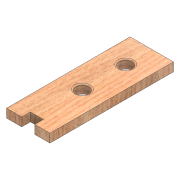
# Autodesk Inventor part: EndaHaldarar
Saved by Autodesk Inventor 2018 (Build 220112000, 112)
## iProperties
Created: 2020-03-01
Part Number: EndaHaldarar
Material: Wood (Birch)
Document SubType Name: Modeling
Designer: Spark
Density: 0.55 g/cm^3
Appearance: Birch - Natural Polished
Author: Spark
Autodesk Inventor part; units mm, degrees
ref_plane "YZ Plane" through (0, 0, 0) normal (1, 0, 0) x (0, 1, 0)
ref_plane "XZ Plane" through (0, 0, 0) normal (0, 1, 0) x (-1, 0, 0)
ref_plane "XY Plane" through (0, 0, 0) normal (0, 0, 1) x (1, 0, 0)
sketch "Sketch1" plane through (0, 0, 0) normal (0, 0, 1) x (1, 0, 0)
  line L0 (0, 0) -> (100, 0)
  line L1 (100, 0) -> (100, 285)
  line L2 (100, 285) -> (0, 285)
  line L3 (0, 285) -> (0, 0)
  dimension "d0" = 100
  dimension "d1" = 285
  constraints: 8 end point, 2 parallel, 1 horizontal, 1 perpendicular
  measures "d0" distance of L2.end L1.end
  measures "d1" distance of L0.end L1.end
extrude "Extrusion1" add sketch "Sketch1" along normal blind 20
sketch "Sketch2" plane through (0, 0, 0) normal (0, 0, -1) x (-1, 0, 0)
  circle A0 centre (-50, 125) radius 15
  circle A1 centre (-50, 225) radius 15
  line L0 (0, 285) -> (0, 0) projected
  line L1 (0, 0) -> (-100, 0) projected
  line L2 (-100, 285) -> (0, 285) projected
  dimension "d5" = 30
  dimension "d6" = 50
  dimension "d7" = 50
  dimension "d9" = 100
  dimension "d17" = 60
  constraints: 2 centre point, 1 equal radius
  measures "d5" diameter of A0
  measures "d6" distance from line of L0 A1.centre
  measures "d7" distance from line of L0 A0.centre
  measures "d9" distance of A1.centre A0.centre
  measures "d17" distance from line of L2 A1.centre
extrude "Extrusion2" cut sketch "Sketch2" against normal up to next
sketch "Sketch3" plane through (0, 0, 0) normal (0, 0, -1) x (-1, 0, 0)
  line L0 (0, 0) -> (-100, 0) projected
  line L1 (-35, 0) -> (-35, 20)
  line L2 (-35, 20) -> (-65, 20)
  line L3 (-65, 20) -> (-65, 0)
  line L4 (0, 285) -> (0, 0) projected
  dimension "d12" = 20
  dimension "d13" = 30
  dimension "d14" = 35
  constraints: 6 end point, 2 perpendicular, 2 point on line, 1 vertical
  measures "d12" distance of L1.start L1.end
  measures "d13" distance between parallel lines of L1 L3
  measures "d14" distance between parallel lines of L4 L1
extrude "Extrusion3" cut sketch "Sketch3" against normal up to next
sketch "Sketch4" plane through (0, 0, 0) normal (-1, 0, 0) x (0, 0, 1)
  line L0 (0, 285) -> (0, 0) projected
  line L1 (0, 0) -> (20, 0) projected
  line L2 (20, 285) -> (20, 0) projected
  line L3 (0, 285) -> (20, 285) projected
  line L4 (20, 285) -> (90.7107, 214.2893) construction
  line L5 (20, 285) -> (120, 285) construction
  dimension "d18" = 100
  dimension "d19" = 45
  constraints: 4 end point, 1 equal length, 1 horizontal
  measures "d18" distance of L2.start L4.end
  measures "d19" angle of L4 L5
fillet "Fillet3" radius 3 2 edges at (65, 125, 20) (65, 225, 20)
body "Solid1"
